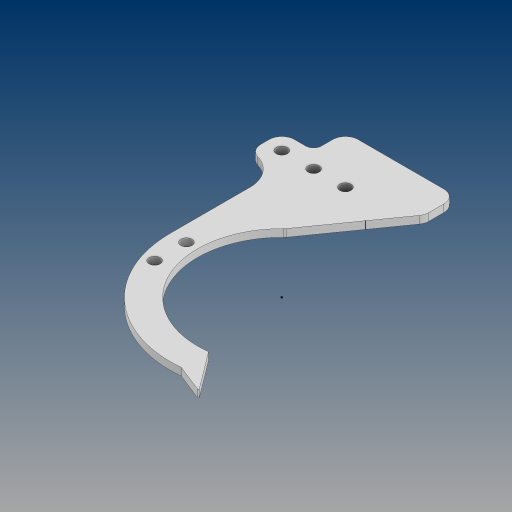
# Autodesk Inventor part: Climb hook
Saved by Autodesk Inventor 2023 (Build 270158000, 158)
## iProperties
Created: 2023-08-23
Part Number: Climb hook
Material: Generic
Document SubType Name: Modeling
Designer: eddie
Density: 1 g/cm^3
Appearance: Default
Author: eddie
## iProperties of the stored document Climb hook_3DPrint.ipt
Created: 2023-08-23
Part Number: Climb hook_3DPrint
Material: Generic
Document SubType Name: Modeling
Designer: eddie
Density: 1 g/cm^3
Appearance: Default
Author: eddie
Autodesk Inventor part; units mm, degrees
ref_plane "YZ Plane" through (0, 0, 0) normal (1, 0, 0) x (0, 1, 0)
ref_plane "XZ Plane" through (0, 0, 0) normal (0, 1, 0) x (-1, 0, 0)
ref_plane "XY Plane" through (0, 0, 0) normal (0, 0, 1) x (1, 0, 0)
sketch "Sketch1" plane through (0, 0, 0) normal (0, 1, 0) x (-1, 0, 0)
  circle A0 centre (0, 0) radius 33.655
  circle A1 centre (0, 0) radius 44.45
  line L0 (0, 44.45) -> (0, 33.655)
  line L1 (7.4782, -32.8136) -> (9.9419, -43.3239)
  line L2 (0, -44.45) -> (44.45, 0)
  line L3 (0, -44.45) -> (0, -69.85)
  line L4 (0, -69.85) -> (38.1, -69.85) construction
  line L5 (-4.1275, 44.258) -> (-4.1275, 33.4009)
  line L6 (-4.1275, 44.258) -> (-15.6469, 48.7936)
  line L7 (-15.6469, 48.7936) -> (-4.1275, 33.4009)
  line L8 (0, -69.85) -> (44.45, -69.85)
  line L9 (44.45, -69.85) -> (44.45, 0)
  line L10 (44.45, -69.85) -> (69.85, -69.85)
  line L11 (69.85, -69.85) -> (69.85, -44.45)
  line L12 (69.85, -44.45) -> (44.45, -44.45)
  line L13 (69.85, -44.45) -> (69.85, -50.8)
  line L14 (69.85, -50.8) -> (63.5, -50.8)
  circle A2 centre (63.5, -50.8) radius 2.2225
  line L15 (63.5, -50.8) -> (50.8, -50.8)
  circle A3 centre (50.8, -50.8) radius 2.2225
  line L16 (50.8, -50.8) -> (50.8, -63.5)
  circle A4 centre (50.8, -63.5) radius 2.2225
  line L17 (50.8, -63.5) -> (63.5, -63.5)
  circle A5 centre (63.5, -63.5) radius 2.2225
  line L18 (44.45, 0) -> (38.1, 0)
  circle A6 centre (38.1, 0) radius 2.2225
  line L19 (38.1, 0) -> (38.1, 12.7)
  circle A7 centre (38.1, 12.7) radius 2.2225
  line L20 (57.15, -69.85) -> (57.15, -44.45)
  line L21 (0, -57.15) -> (30.7326, -13.7174)
  line L22 (0, -57.15) -> (69.85, -57.15)
  line L23 (50.8, -50.8) -> (38.1, -50.8)
  circle A8 centre (38.1, -50.8) radius 2.2225
  line L24 (38.1, -50.8) -> (25.4, -50.8)
  circle A9 centre (25.4, -50.8) radius 2.2225
  point P0 (13.7174, -30.7326)
  point P1 (30.7326, -13.7174)
  point P2 (-11.3028, 42.9889)
  point P3 (23.1613, -24.4175)
  point P4 (9.9025, -43.1554)
  point P5 (9.7529, -43.3669)
  point P6 (57.15, -57.15)
  point P7 (44.45, -57.15)
  dimension "d0" = 67.31
  dimension "d1" = 88.9
  dimension "d23" = 44.45
  dimension "d24" = 6.35
  dimension "d25" = 6.35
  dimension "d26" = 4.445
  dimension "d27" = 12.7
  dimension "d28" = 4.445
  dimension "d29" = 12.7
  dimension "d30" = 4.445
  dimension "d31" = 12.7
  dimension "d32" = 4.445
  dimension "d35" = 6.35
  dimension "d36" = 4.445
  dimension "d37" = 12.7
  dimension "d38" = 4.445
  dimension "d47" = 12.7
  dimension "d48" = 4.445
  dimension "d49" = 12.7
  dimension "d50" = 4.445
  constraints: 50 end point, 10 centre point, 10 point on circle, 9 coincident, 6 horizontal, 5 point on line, 4 midpoint, 4 vertical, 3 perpendicular
  measures "d0" diameter of A0
  measures "d1" diameter of A1
  measures "d23" distance of L3.end L8.end
  measures "d24" distance of L11.end L13.end
  measures "d25" distance of L13.end L14.end
  measures "d26" diameter of A2
  measures "d27" distance of L15.start L15.end
  measures "d28" diameter of A3
  measures "d29" distance of L16.start L16.end
  measures "d30" diameter of A4
  measures "d31" distance of L17.start L17.end
  measures "d32" diameter of A5
  measures "d35" distance of L9.end L18.end
  measures "d36" diameter of A6
  measures "d37" distance of L19.start L19.end
  measures "d38" diameter of A7
  measures "d47" distance of L16.start L23.end
  measures "d48" diameter of A8
  measures "d49" distance of L24.start L24.end
  measures "d50" diameter of A9
extrude "Extrusion1" add sketch "Sketch1" along normal blind 3 contours A0 L0 A1 L2 | A0 L5 A1 L0 | L2 A1 L1 L21 A0 | L7 A1 L5 | L9 L22 L21 A1 | A1 L7 L6 | L12 L20 L15 A3 L23 L9 | L23 A3 L16 L22 L9 | L22 L9 L8 L3 | L20 L22 L16 A3 L15
sketch "Sketch3" plane through (0, 3, 0) normal (0, 1, 0) x (1, 0, 0)
  point P0 (0, 0)
fillet "Fillet3" radius 0.254 1 edges at (15.6469, 1.5, 48.7936)
fillet "Fillet5" radius 12.7 1 edges at (-44.45, 1.5, -44.45)
sketch "Sketch4" plane through (0, 3, 0) normal (0, 1, 0) x (1, 0, 0)
  point P0 (0, 0)
fillet "Fillet9" radius 5.08 1 edges at (0, 1.5, -69.85)
fillet "Fillet10" radius 5.08 1 edges at (0, 1.5, -57.15)
fillet "Fillet11" radius 5.08 1 edges at (-23.1613, 1.5, -24.4175)
fillet "Fillet12" radius 5.08 2 edges at (-57.1495, 1.5, -44.45) (-57.15, 1.5, -44.45)
fillet "Fillet14" radius 5.08 1 edges at (-57.15, 1.5, -57.15)
fillet "Fillet15" radius 5.08 1 edges at (-44.45, 1.5, -69.85)
fillet "Fillet16" radius 3.175 1 edges at (-44.45, 1.5, -57.15)
body "Solid1"
